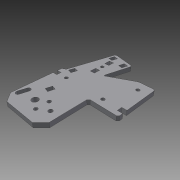
# Autodesk Inventor part: z_axis_top
Saved by Autodesk Inventor 2014 (Build 180170000, 170)
## iProperties
Created: 2013-12-06
Part Number: z_axis_top
Material: Generic
Document SubType Name: Modeling
Designer: buben
Density: 1 g/cm^3
Appearance: Default
Author: buben
Subject: Laser Cutted
Autodesk Inventor part; units mm, degrees
ref_plane "YZ Plane" through (0, 0, 0) normal (1, 0, 0) x (0, 1, 0)
ref_plane "XZ Plane" through (0, 0, 0) normal (0, 1, 0) x (-1, 0, 0)
ref_plane "XY Plane" through (0, 0, 0) normal (0, 0, 1) x (1, 0, 0)
sketch "Sketch1" plane through (0, 0, 0) normal (0, 0, 1) x (1, 0, 0)
  line L0 (0, 0) -> (0, -52)
  line L1 (0, -52) -> (10, -62)
  line L2 (10, -62) -> (50, -62)
  line L3 (50, -62) -> (60, -52)
  line L4 (60, -52) -> (60, -6)
  line L5 (0, 0) -> (6, 0)
  line L6 (6, 0) -> (6, 6)
  line L7 (6, 6) -> (0, 6)
  line L8 (0, 6) -> (0, 12)
  line L9 (0, 12) -> (76, 50)
  line L10 (60, -6) -> (96, -6)
  line L11 (96, -6) -> (96, 0)
  line L12 (96, 0) -> (90, 0)
  line L13 (90, 0) -> (90, 6)
  line L14 (90, 6) -> (96, 6)
  line L15 (96, 6) -> (96, 50)
  line L16 (96, 50) -> (76, 50)
  circle A0 centre (49, -42) radius 2.5
  circle A1 centre (26, -42) radius 4
  dimension "d0" = 45
  dimension "d1" = 10
  dimension "d2" = 8
  dimension "d3" = 5
  dimension "d4" = 23
  dimension "d5" = 6
  dimension "d6" = 6
  dimension "d7" = 6
  dimension "d8" = 42
  dimension "d9" = 6
  dimension "d10" = 26
  dimension "d11" = 44
  dimension "d12" = 20
  dimension "d14" = 6
  dimension "d15" = 84
  dimension "d16" = 60
  dimension "d17" = 20
  constraints: 34 end point, 7 parallel, 5 collinear, 5 perpendicular, 2 centre point, 2 horizontal alignment, 1 vertical
  measures "d0" angle of L0 L1
  measures "d1" horizontal distance of L1.end L0.end
  measures "d2" diameter of A1
  measures "d3" diameter of A0
  measures "d4" distance of A1.centre A0.centre
  measures "d5" distance of L5.end L6.end
  measures "d6" distance of L0.start L5.end
  measures "d7" distance of L13.end L14.end
  measures "d8" distance from line of A1.centre L5
  measures "d9" distance of L10.end L11.end
  measures "d10" distance from line of A1.centre L0
  measures "d11" distance of L14.end L15.end
  measures "d12" distance of L15.end L9.end
  measures "d14" distance of L7.end L8.end
  measures "d15" distance between parallel lines of L13 L6
  measures "d16" distance between parallel lines of L4 L0
  measures "d17" distance from line of L2 A1.centre
extrude "Extrusion1" add sketch "Sketch1" along normal blind 6
chamfer "Chamfer1" distance 2 angle 45 3 edges at (60, -6, 3) (96, 50, 3) (96, -6, 3)
sketch "Sketch2" plane through (0, 0, 6) normal (0, 0, 1) x (1, 0, 0)
  line L0 (96, 6) -> (96, 48) projected
  line L1 (94, 50) -> (76, 50) projected
  circle A0 centre (84, 38) radius 2.25
  circle A1 centre (84, 38) radius 4.5 construction
  dimension "d23" = 4.5
  dimension "d24" = 12
  dimension "d25" = 9
  dimension "d26" = 12
  constraints: 2 centre point, 1 coincident
  measures "d23" diameter of A0
  measures "d24" distance from line of L0 A0.centre
  measures "d25" diameter of A1
  measures "d26" distance from line of L1 A0.centre
extrude "Extrusion2" cut sketch "Sketch2" against normal through all
sketch "Sketch3" plane through (0, 0, 6) normal (0, 0, 1) x (1, 0, 0)
  circle A0 centre (84, 38) radius 2.25 projected
  line L0 (94, 50) -> (76, 50) projected
  line L1 (0, 12) -> (0, 6) projected
  line L2 (0, 0) -> (0, -52) projected
  line L3 (10, -62) -> (50, -62) projected
  line L4 (62, -6) -> (94, -6) projected
  circle A1 centre (6.5, -42) radius 2 construction
  line L5 (81, 50) -> (81, -6) construction
  line L6 (0, 9) -> (81, 9) construction
  line L7 (40.5, 9) -> (40.5, 90) construction
  line L8 (40.5, 90) -> (6.5, -42) construction
  line L9 (7.7472, -37.158) -> (5.2528, -46.842) construction
  line L10 (4.842, -36.4097) -> (2.3477, -46.0937)
  line L11 (8.158, -47.5903) -> (10.6523, -37.9063)
  arc A2 (10.6523, -37.9063) -> (4.842, -36.4097) centre (7.7472, -37.158) ccw
  arc A3 (2.3477, -46.0937) -> (8.158, -47.5903) centre (5.2528, -46.842) ccw
  point P0 (6.5, -42)
  dimension "d29" = 20
  dimension "d30" = 6.5
  dimension "d31" = 4
  dimension "d32" = 3
  dimension "d33" = 10
  dimension "d34" = 6
  constraints: 16 end point, 4 perpendicular, 4 point on circle, 4 tangent, 3 centre point, 3 midpoint, 3 point on line, 2 parallel, 1 coincident
  measures "d29" distance from line of L3 L8.end
  measures "d30" distance from line of L2 L8.end
  measures "d31" diameter of A1
  measures "d32" distance from line of L5 A0.centre
  measures "d33" distance of L9.start L9.end
  measures "d34" distance between parallel lines of L10 L11
extrude "Extrusion3" cut sketch "Sketch3" against normal through all contours A2 L11 A3 L10
sketch "Sketch4" plane through (0, 0, 6) normal (0, 0, 1) x (1, 0, 0)
  arc A0 (2.3477, -46.0937) -> (8.158, -47.5903) centre (5.2528, -46.842) ccw projected
  line L0 (2.3477, -46.0937) -> (4.842, -36.4097) projected
  arc A1 (10.6523, -37.9063) -> (4.842, -36.4097) centre (7.7472, -37.158) ccw projected
  circle A2 centre (84, 38) radius 2.25 projected
  line L1 (94, 50) -> (76, 50) projected
  line L2 (76, 50) -> (0, 12) projected
  line L3 (0, 12) -> (0, 6) projected
  line L4 (62, -6) -> (94, -6) projected
  line L5 (81, 50) -> (81, -6) construction
  line L6 (0, 9) -> (81, 9) construction
  line L7 (40.5, 9) -> (40.5, 90) construction
  line L8 (40.5, 90) -> (7.7472, -37.158) construction
  line L9 (25.2478, 93.9286) -> (-7.505, -33.2295) construction
  line L10 (55.7522, 86.0714) -> (22.9993, -41.0866) construction
  line L11 (25.2478, 93.9286) -> (55.7522, 86.0714) construction
  line L12 (-7.505, -33.2295) -> (22.9993, -41.0866) construction
  line L13 (7.7472, -37.158) -> (5.2528, -46.842) construction
  line L14 (21.2558, 78.4302) -> (51.7602, 70.573)
  line L15 (21.2558, 78.4302) -> (4.7578, 14.3789)
  line L16 (51.7602, 70.573) -> (42.0944, 33.0472)
  line L17 (4.7578, 14.3789) -> (42.0944, 33.0472)
  point P0 (6.5, -42)
  point P1 (10.492, -26.5016)
  point P2 (36.508, 74.5016)
  dimension "d37" = 3
  dimension "d38" = 31.5
  dimension "d39" = 15.75
  dimension "d40" = 136.3085
  dimension "d41" = 104.3
  dimension "d52" = 16.0042
  constraints: 26 end point, 11 point on line, 8 perpendicular, 6 midpoint, 2 parallel, 1 collinear
  measures "d37" distance from line of L5 A2.centre
  measures "d38" distance between parallel lines of L10 L9
  measures "d39" distance from line of L8 L9.end
  measures "d40" distance of point (6.5, -42) L7.end
  measures "d41" distance of point (10.492, -26.502) point (36.508, 74.502)
  measures "d52" distance between parallel lines of L14 L11
extrude "Extrusion4" add sketch "Sketch4" against normal blind 6 contours L2 L15 L14 L16
sketch "Sketch6" plane through (0, 0, 6) normal (0, 0, 1) x (1, 0, 0)
  line L0 (42.0944, 33.0472) -> (51.7602, 70.573) projected
  line L1 (51.7602, 70.573) -> (21.2558, 78.4302) projected
  line L2 (47.8573, 67.4478) -> (42.0469, 68.9444)
  line L3 (42.0469, 68.9444) -> (40.0514, 61.1972)
  line L4 (40.0514, 61.1972) -> (45.8618, 59.7006)
  line L5 (45.8618, 59.7006) -> (47.8573, 67.4478)
  line L6 (25.8322, -18.0612) -> (20.0219, -16.5646)
  line L7 (20.0219, -16.5646) -> (18.0264, -24.3117)
  line L8 (18.0264, -24.3117) -> (23.8367, -25.8083)
  line L9 (23.8367, -25.8083) -> (25.8322, -18.0612)
  dimension "d53" = 8
  dimension "d54" = 6
  dimension "d55" = 8
  dimension "d56" = 4
  dimension "d57" = 3
  dimension "d58" = 80.3
  constraints: 16 end point, 6 parallel, 2 collinear, 2 perpendicular
  measures "d53" distance of L4.end L2.start
  measures "d54" distance of L2.start L2.end
  measures "d55" distance of L8.end L6.start
  measures "d56" distance between parallel lines of L1 L2
  measures "d57" distance between parallel lines of L0 L5
  measures "d58" distance between parallel lines of L6 L4
extrude "Extrusion5" cut sketch "Sketch6" against normal through all
sketch "Sketch7" plane through (0, 0, 6) normal (0, 0, 1) x (1, 0, 0)
  line L0 (42.0469, 68.9444) -> (47.8573, 67.4478) projected
  line L1 (21.2558, 78.4302) -> (4.7578, 14.3789) projected
  line L2 (28.9736, 72.3117) -> (23.1633, 73.8083)
  line L3 (23.1633, 73.8083) -> (21.1678, 66.0612)
  line L4 (21.1678, 66.0612) -> (26.9781, 64.5646)
  line L5 (26.9781, 64.5646) -> (28.9736, 72.3117)
  line L6 (15.7536, 20.987) -> (9.9432, 22.4836)
  line L7 (9.9432, 22.4836) -> (7.9478, 14.7365)
  line L8 (7.9478, 14.7365) -> (13.7581, 13.2398)
  line L9 (13.7581, 13.2398) -> (15.7536, 20.987)
  line L10 (13.7581, 13.2398) -> (7.9478, 14.7365) construction
  line L11 (7.9478, 14.7365) -> (2.2108, -7.5366) construction
  line L12 (2.2108, -7.5366) -> (8.0211, -9.0332) construction
  line L13 (8.0211, -9.0332) -> (13.7581, 13.2398) construction
  dimension "d61" = 8
  dimension "d62" = 6
  dimension "d63" = 3
  dimension "d64" = 45
  dimension "d65" = 23
  constraints: 24 end point, 11 equal length, 3 collinear, 3 perpendicular
  measures "d61" distance of L2.end L3.end
  measures "d62" distance of L2.start L2.end
  measures "d63" distance between parallel lines of L1 L3
  measures "d64" distance between parallel lines of L6 L4
  measures "d65" distance of L7.end L11.end
extrude "Extrusion6" cut sketch "Sketch7" against normal through all
sketch "Sketch8" plane through (0, 0, 6) normal (0, 0, 1) x (1, 0, 0)
  line L0 (15.7536, 20.987) -> (13.7581, 13.2398) projected
  line L1 (18.0264, -24.3117) -> (20.0219, -16.5646) projected
  line L2 (90, 0) -> (90, 6) projected
  line L3 (6, 6) -> (6, 0) projected
  circle A0 centre (18.0909, 3) radius 2.25
  circle A1 centre (70, 3) radius 2.25
  line L4 (6, 3) -> (90, 3) construction
  dimension "d68" = 4.5
  dimension "d69" = 13.5
  dimension "d70" = 6.75
  dimension "d71" = 20
  constraints: 2 centre point, 2 end point, 2 midpoint, 2 point on line, 1 equal radius
  measures "d68" diameter of A0
  measures "d69" distance between parallel lines of L0 L1
  measures "d70" distance from line of L0 A0.centre
  measures "d71" distance from line of L2 A1.centre
extrude "Extrusion7" cut sketch "Sketch8" against normal through all
sketch "Sketch9" plane through (0, 0, 6) normal (0, 0, 1) x (1, 0, 0)
  line L0 (28.9736, 72.3117) -> (26.9781, 64.5646) projected
  line L1 (40.0514, 61.1972) -> (42.0469, 68.9444) projected
  line L2 (0, 6) -> (6, 6) projected
  circle A0 centre (29.1667, 46) radius 2.25
  line L3 (0, 12) -> (0, 6) projected
  dimension "d74" = 4.5
  dimension "d75" = 13.5
  dimension "d76" = 6.75
  dimension "d77" = 40
  dimension "d90" = 29.1667
  constraints: 1 centre point
  measures "d74" diameter of A0
  measures "d75" distance between parallel lines of L1 L0
  measures "d76" distance from line of A0.centre L0
  measures "d77" distance from line of L2 A0.centre
  measures "d90" distance from line of A0.centre L3
extrude "Extrusion8" cut sketch "Sketch9" against normal through all
chamfer "Chamfer2" distance 2 angle 45 3 edges at (21.2558, 78.4302, 3) (51.7602, 70.573, 3) (42.0944, 33.0472, 3)
sketch "Sketch11" plane through (0, 0, 6) normal (0, 0, 1) x (1, 0, 0)
  circle A0 centre (29.1667, 46) radius 2.25 projected
  line L0 (26.1667, 61.5) -> (32.1667, 61.5)
  line L1 (32.1667, 61.5) -> (32.1667, 53.5)
  line L2 (32.1667, 53.5) -> (26.1667, 53.5)
  line L3 (26.1667, 53.5) -> (26.1667, 61.5)
  line L4 (26.1667, 38.5) -> (32.1667, 38.5)
  line L5 (32.1667, 38.5) -> (32.1667, 30.5)
  line L6 (32.1667, 30.5) -> (26.1667, 30.5)
  line L7 (26.1667, 30.5) -> (26.1667, 38.5)
  line L8 (32.1667, 53.5) -> (26.1667, 38.5) construction
  line L9 (32.1667, 38.5) -> (26.1667, 53.5) construction
  dimension "d84" = 8
  dimension "d85" = 6
  dimension "d86" = 8
  dimension "d87" = 15
  constraints: 20 end point, 4 parallel, 2 collinear, 2 horizontal, 2 perpendicular, 1 coincident, 1 midpoint
  measures "d84" distance of L2.end L0.start
  measures "d85" distance of L0.start L0.end
  measures "d86" distance of L6.end L4.start
  measures "d87" distance between parallel lines of L4 L2
extrude "Extrusion9" cut sketch "Sketch11" against normal through all contours L0 L1 L2 L3 | L4 L5 L6 L7
sketch "Sketch12" plane through (0, 0, 6) normal (0, 0, 1) x (1, 0, 0)
  line L0 (94, 50) -> (76, 50) projected
  circle A0 centre (26, -42) radius 4 projected
  circle A1 centre (49, -42) radius 2.5 projected
  circle A2 centre (37.5, -34.5) radius 2.25
  circle A3 centre (37.5, -49.5) radius 2.25
  line L1 (26, -42) -> (49, -42) construction
  line L2 (37.5, -34.5) -> (37.5, -49.5) construction
  point P0 (37.5, -42)
  dimension "d91" = 15
  dimension "d92" = 4.5
  constraints: 4 end point, 2 centre point, 2 midpoint, 1 equal radius, 1 parallel, 1 perpendicular, 1 vertical alignment
  measures "d91" distance of L2.start L2.end
  measures "d92" diameter of A2
extrude "Extrusion10" cut sketch "Sketch12" against normal through all contours A2 | A3
equation "\"d39\" = 0.5 * d38"
equation "\"d52\" = -0.5 * d41 + 0.5 * d40"
equation "\"d70\" = 0.5 * d69"
equation "\"d76\" = 0.5 * d75"
body "Solid1"
